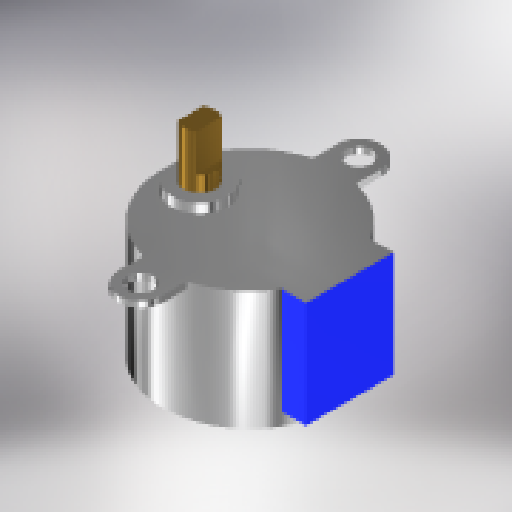
# Autodesk Inventor part: 28BYJ-48
Saved by Autodesk Inventor 2023 (Build 270158000, 158)
## iProperties
Created: 2022-05-01
Part Number: 28BYJ-48
Material: Aluminum 6061
Document SubType Name: Modeling
Designer: Remo
Density: 2.7 g/cm^3
Appearance: Aluminum - Flat
Mass: 35.2283 g
Surface Area: 35.4077 cm^2
Volume: 13.0475 cm^3
Author: Remo
Autodesk Inventor part; units mm, degrees
ref_plane "YZ Plane" through (0, 0, 0) normal (1, 0, 0) x (0, 1, 0)
ref_plane "XZ Plane" through (0, 0, 0) normal (0, 1, 0) x (-1, 0, 0)
ref_plane "XY Plane" through (0, 0, 0) normal (0, 0, 1) x (1, 0, 0)
sketch "Sketch1" plane through (0, 0, 0) normal (0, 1, 0) x (-1, 0, 0)
  circle A0 centre (0, 0) radius 14
  dimension "d0" = 28
  constraints: 1 centre point, 1 coincident
  measures "d0" diameter of A0
extrude "Extrusion1" add sketch "Sketch1" along normal blind 19
sketch "Sketch3" plane through (0, 19, 0) normal (0, 1, 0) x (1, 0, 0)
  circle A0 centre (0, 0) radius 14 projected
  line L0 (3.5, 13.5554) -> (3.5, 17.5) projected
  arc A1 (3.5, 17.5) -> (-3.5, 17.5) centre (0, 17.5) ccw projected
  line L1 (-3.5, 17.5) -> (-3.5, 13.5554) projected
  arc A2 (3.5, 13.5554) -> (-3.5, 13.5554) centre (0, 0) ccw projected
  circle A3 centre (0, 17.5) radius 2 projected
  line L2 (-3.5, -13.5554) -> (-3.5, -17.5) projected
  arc A4 (-3.5, -17.5) -> (3.5, -17.5) centre (0, -17.5) ccw projected
  line L3 (3.5, -17.5) -> (3.5, -13.5554) projected
  arc A5 (-3.5, -13.5554) -> (3.5, -13.5554) centre (0, 0) ccw projected
  circle A6 centre (0, -17.5) radius 2 projected
  circle A7 centre (-8, 0) radius 4.5
  dimension "d8" = 9
  dimension "d9" = 8
  constraints: 1 centre point
  measures "d8" diameter of A7
  measures "d9" distance of point (0, 0) A7.centre
extrude "Extrusion3" add sketch "Sketch3" along normal blind 1.5 contours A7
sketch "Sketch4" plane through (-8, 20.5, 0) normal (0, 1, 0) x (1, 0, 0)
  circle A0 centre (0, 0) radius 4.5 projected
  circle A1 centre (0, 0) radius 2.5
  point P0 (8, 0)
  dimension "d12" = 5
  constraints: 1 centre point, 1 coincident
  measures "d12" diameter of A1
extrude "Extrusion4" add sketch "Sketch4" along normal blind 8.5 contours A1
sketch "Sketch5" plane through (-8, 29, 0) normal (0, 1, 0) x (1, 0, 0)
  circle A0 centre (0, 0) radius 2.5 projected
  circle A1 centre (0, 0) radius 2.5 projected
  line L0 (-1.5, 2) -> (-1.5, -2)
  line L1 (1.5, -2) -> (1.5, 2)
  point P0 (8, 0)
  point P1 (1.5, 2)
  point P2 (1.5, -2)
  dimension "d15" = 1.5
  dimension "d16" = 3
  constraints: 4 end point, 4 point on circle, 1 vertical
  measures "d15" distance from line of L0 A0.centre
  measures "d16" distance between parallel lines of L0 L1
extrude "Extrusion5" cut sketch "Sketch5" against normal blind 6 contours A0 L1 | L0 A0
sketch "Sketch7" plane through (0, 19, 0) normal (0, 1, 0) x (1, 0, 0)
  circle A0 centre (-8, 0) radius 4.5 projected
  circle A1 centre (0, 0) radius 14 projected
  line L0 (0, -17.5) -> (0, 17.5) construction
  line L1 (3.5, -17.5) -> (3.5, 17.5)
  line L2 (-3.5, 17.5) -> (-3.5, -17.5)
  arc A2 (-3.5, -17.5) -> (3.5, -17.5) centre (0, -17.5) ccw
  arc A3 (3.5, 17.5) -> (-3.5, 17.5) centre (0, 17.5) ccw
  circle A4 centre (0, 17.5) radius 2
  circle A5 centre (0, -17.5) radius 2
  point P0 (3.5, -13.5554)
  point P1 (-3.5, -13.5554)
  point P2 (-3.5, 13.5554)
  point P3 (3.5, 13.5554)
  dimension "d24" = 35
  dimension "d25" = 3.5
  dimension "d26" = 4
  constraints: 8 end point, 4 centre point, 4 point on circle, 4 tangent, 2 coincident, 1 equal radius, 1 midpoint, 1 parallel, 1 vertical
  measures "d24" distance of L0.start L0.end
  measures "d25" radius of A3
  measures "d26" diameter of A5
extrude "Extrusion7" add sketch "Sketch7" against normal blind 1 contours L2 A3 L1 A1 | A1 L1 A2 L2
sketch "Sketch8" plane through (0, 19, 0) normal (0, 1, 0) x (1, 0, 0)
  arc A0 (3.5, -13.5554) -> (3.5, 13.5554) centre (0, 0) ccw projected
  line L0 (12.1244, 7) -> (16, 7)
  line L1 (16, 7) -> (16, -7)
  line L2 (16, -7) -> (12.1244, -7)
  circle A1 centre (0, 0) radius 14 projected
  point P0 (14.0622, 7)
  point P1 (16, 0)
  point P2 (14, 0)
  dimension "d29" = 7
  dimension "d30" = 7
  dimension "d31" = 2
  constraints: 6 end point, 3 point on circle, 2 midpoint, 2 perpendicular, 1 horizontal
  measures "d29" distance from line of L2 point (0, 0)
  measures "d30" vertical distance of point (0, 0) point (14.062, 7)
  measures "d31" distance of point (16, 0) point (14, 0)
extrude "Extrusion8" add sketch "Sketch8" against normal blind 17 contours A0 L0 L1 L2
equation "\"d16\" = 2 * d15"
equation "\"d30\" = d29"
body "Solid1"
